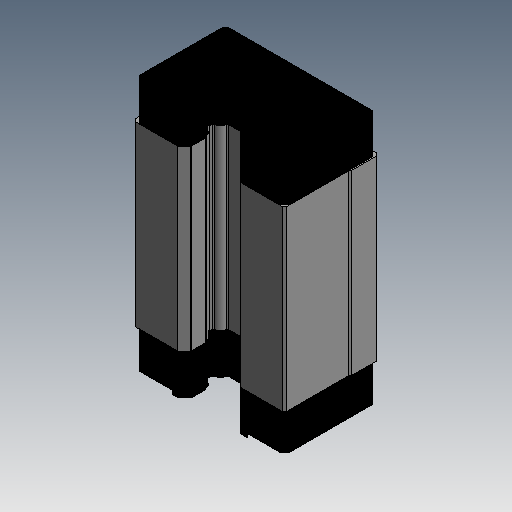
# Autodesk Inventor part: C-SXR24-R_b
Saved by Autodesk Inventor 2020 (Build 240168000, 168)
## iProperties
Part Number: C-SXR24-R_b
Material: 一般
Catalog Web Link: www.cadenas.de
Description: C-SXR, C-SX2R, C-SXRL, C-SX2RL_block-C-VALUE Linear Guides for Heavy Load
Vendor: MISUMI
Document SubType Name: Modeling
Designer: partserver
Manufacturer: MISUMI
Mass: 31.9411 g
Surface Area: 88.9166 cm^2
Volume: 31.9411 cm^3
Density: 1 g/cm^3
Appearance: PSOLRGB-192-192-192
Category: PARTsolutions
Company: MISUMI
PSOL_IDENT_0: {$CADENAS_DATA\23d-libs\misumi\metric\06_linear_guides\06_cn\c_sxr\c_sxr_block.prj},199 {VTYP=3D},{N
PSOL_IDENT_1: B=C-SXR24-R_b},{LINA=C-SXR24-R},{NN=C-SXR, C-SX2R, C-SXRL, C-SX2RL_block},{DATE=20.05.2021 06:43:21}
PSOL_IDENT_2: ,{GEOMDATE=17.04.2020 08:25:00},{VERSION=},{LINEID=10},{WBVAR=NOB,LT,BD},{WBNUMERIC=}  {NB=C-SXR24-R
PSOL_IDENT_3: _b},{LINA=C-SXR24-R},{KT=DUMMY},{PN=C-SXR24-R},{TYPE=C-SX},{H=24},{NOB=},{LT=},{W=34},{L1=55.9},{B=2
PSOL_IDENT_4: 6},{C=26},{SLL=M4x5},{S=4.000},{LL=5.000},{L2=39.5},{K=20.8},{T=6.20},{CBB=0.5},{E=7},{T1=5.5},{H1=1
PSOL_IDENT_5: 3.0},{W1=15},{W2=9.5},{CAA=0.5},{DD1=4.5},{DD2=7.5},{HH=6.0},{LW1=7.217},{LW2=11.000},{LH1=8.221},{L
PSOL_IDENT_6: H2=4.659},{LH3=3.221},{LH4=4.700},{LC1=0.300},{LC2=2.000},{LC3=0.500},{LR1=1.431},{LR2=0.300},{LR3=0
PSOL_IDENT_7: .300},{LR4=0.300},{BW=11.000},{BW2=33.400},{BH=20.250},{BH2=0.300},{BA1=149.392},{BA2=151.695},{CBB2=
PSOL_IDENT_8: 0.750},{CBB3=0.500},{CBB4=1.000},{HL=7.100},{BW3=7.105},{BW4=13.000},{BW5=17.000},{BW6=0.250},{BH3=1
PSOL_IDENT_9: 0.750},{BH4=2.417},{BH5=2.188},{BH6=0.500},{BA3=119.244},{BA4=131.813},{BA5=135.000},{BT=0.800},{BR=
PSOL_IDENT_10: 1.000},{BD=R}
NB: C-SXR24-R_b
NN: C-SXR, C-SX2R, C-SXRL, C-SX2RL_block
NT: C-VALUE Linear Guides for Heavy Load
NBSYN: $PN._b
LINA: C-SXR24-R
CATALOG: Misumi
PN: C-SXR24-R
H: 24
NOB: 1
LT: Selectable
W: 34
L1: 55.9
B: 26
C: 26
SLL: M4x5
L2: 39.5
K: 20.8
T: 6.2
CBB: 0.5
E: 7
T1: 5.5
BD: R
SUPPLIER: MISUMI
ARTICLENO: C-SXR24-R_b
BOMINFO: C-SXR24-R
CREATOR: CADENAS GmbH
Title: C-SXR24-R
Author: Cadenas PARTsolutions
Comments: C-VALUE Linear Guides for Heavy Load
Autodesk Inventor part; units mm, degrees
sketch "Sketch_1" plane through (0, 0, 0) normal (0, 0, 1) x (1, 0, 0)
  line L0 (-17, 23.5) -> (-17, 17.8)
  line L1 (-17, 17.8) -> (-16.75, 17.3358)
  line L2 (-16.75, 17.3358) -> (-16.75, 3.7)
  line L3 (-16.75, 3.7) -> (-16.25, 3.2)
  line L4 (-16.25, 3.2) -> (16.5, 3.2)
  line L5 (16.5, 3.2) -> (17, 3.7)
  line L6 (17, 3.7) -> (17, 23.5)
  line L7 (17, 23.5) -> (16.5, 24)
  line L8 (16.5, 24) -> (5.5, 24)
  line L9 (5.5, 24) -> (4.9929, 23.7)
  line L10 (4.9929, 23.7) -> (-4.9929, 23.7)
  line L11 (-4.9929, 23.7) -> (-5.5, 24)
  line L12 (-5.5, 24) -> (-16.5, 24)
  line L13 (-16.5, 24) -> (-17, 23.5)
  constraints: 28 end point
extrude "Extrusion1" add sketch "Sketch_1" along normal mid plane 39.5
sketch "Sketch_2" plane through (0, 0, 0) normal (0, 0, 1) x (1, 0, 0)
  line L0 (-16.7, 22.75) -> (-16.7, 4.3)
  line L1 (-16.7, 4.3) -> (-15.7, 3.3)
  line L2 (-15.7, 3.3) -> (15.7, 3.3)
  line L3 (15.7, 3.3) -> (16.7, 4.3)
  line L4 (16.7, 4.3) -> (16.7, 22.75)
  line L5 (16.7, 22.75) -> (15.95, 23.5)
  line L6 (15.95, 23.5) -> (-15.95, 23.5)
  line L7 (-15.95, 23.5) -> (-16.7, 22.75)
  constraints: 16 end point
extrude "Extrusion2" add sketch "Sketch_2" along normal mid plane 55.9
sketch "Sketch_32" plane through (0, 18.5, 0) normal (0, 1, 0) x (1, 0, 0)
  line L0 (0, -27.95) -> (0, -34.95)
  arc A0 (-3, -31.95) -> (0, -34.95) centre (0, -31.95) ccw
  line L1 (-3, -31.95) -> (-3, -27.95)
  line L2 (-3, -27.95) -> (0, -27.95)
  line L3 (0, -27.95) -> (0, -34.95)
  constraints: 8 end point, 2 point on circle, 1 centre point
revolve "Revolution1" add sketch "Sketch_32" angle 360 about axis through (0, 18.5, 27.95) along (0, 0, -1)
sketch "Sketch_33" plane through (0, 0, 27.95) normal (0, 0, 1) x (1, 0, 0)
  circle A0 centre (0, 18.5) radius 3.5
  line L0 (-2.8868, 18.5) -> (-1.4434, 16)
  line L1 (-1.4434, 16) -> (1.4434, 16)
  line L2 (1.4434, 16) -> (2.8868, 18.5)
  line L3 (2.8868, 18.5) -> (1.4434, 21)
  line L4 (1.4434, 21) -> (-1.4434, 21)
  line L5 (-1.4434, 21) -> (-2.8868, 18.5)
  constraints: 12 end point, 1 centre point
extrude "Extrusion3" cut sketch "Sketch_33" along normal blind 7
sketch "Sketch_7" plane through (0, 0, 27.95) normal (0, 0, 1) x (1, 0, 0)
  line L0 (-8.5, 11.2475) -> (-8.5, 9.5386)
  arc A0 (-8.5, 9.5386) -> (-8.1667, 8.7933) centre (-7.5, 9.5386) ccw
  line L1 (-8.1667, 8.7933) -> (-6.8333, 7.6006)
  arc A1 (-6.5, 6.8552) -> (-6.8333, 7.6006) centre (-7.5, 6.8552) ccw
  line L2 (-6.5, 6.8552) -> (-6.5, 5.5286)
  arc A2 (-6.7929, 4.8215) -> (-6.5, 5.5286) centre (-7.5, 5.5286) ccw
  line L3 (-6.7929, 4.8215) -> (-8.3144, 3.3)
  line L4 (-8.3144, 3.3) -> (8.3144, 3.3)
  line L5 (8.3144, 3.3) -> (6.7929, 4.8215)
  arc A3 (6.5, 5.5286) -> (6.7929, 4.8215) centre (7.5, 5.5286) ccw
  line L6 (6.5, 5.5286) -> (6.5, 6.8552)
  arc A4 (6.8333, 7.6006) -> (6.5, 6.8552) centre (7.5, 6.8552) ccw
  line L7 (6.8333, 7.6006) -> (8.1667, 8.7933)
  arc A5 (8.1667, 8.7933) -> (8.5, 9.5386) centre (7.5, 9.5386) ccw
  line L8 (8.5, 9.5386) -> (8.5, 11.2475)
  arc A6 (8.5, 11.2475) -> (8.3725, 11.7361) centre (7.5, 11.2475) ccw
  line L9 (8.3725, 11.7361) -> (7.3914, 13.4885)
  arc A7 (7.3914, 13.4885) -> (6.5188, 14) centre (6.5188, 13) ccw
  line L10 (6.5188, 14) -> (-6.5188, 14)
  arc A8 (-6.5188, 14) -> (-7.3914, 13.4885) centre (-6.5188, 13) ccw
  line L11 (-7.3914, 13.4885) -> (-8.3725, 11.7361)
  arc A9 (-8.3725, 11.7361) -> (-8.5, 11.2475) centre (-7.5, 11.2475) ccw
  constraints: 24 end point, 20 point on circle, 10 centre point
extrude "Extrusion4" add sketch "Sketch_7" along normal blind 0.8
sketch "Sketch_47" plane through (0, 0, -27.95) normal (0, 0, 1) x (1, 0, 0)
  line L0 (-8.5, 11.2475) -> (-8.5, 9.5386)
  arc A0 (-8.5, 9.5386) -> (-8.1667, 8.7933) centre (-7.5, 9.5386) ccw
  line L1 (-8.1667, 8.7933) -> (-6.8333, 7.6006)
  arc A1 (-6.5, 6.8552) -> (-6.8333, 7.6006) centre (-7.5, 6.8552) ccw
  line L2 (-6.5, 6.8552) -> (-6.5, 5.5286)
  arc A2 (-6.7929, 4.8215) -> (-6.5, 5.5286) centre (-7.5, 5.5286) ccw
  line L3 (-6.7929, 4.8215) -> (-8.3144, 3.3)
  line L4 (-8.3144, 3.3) -> (8.3144, 3.3)
  line L5 (8.3144, 3.3) -> (6.7929, 4.8215)
  arc A3 (6.5, 5.5286) -> (6.7929, 4.8215) centre (7.5, 5.5286) ccw
  line L6 (6.5, 5.5286) -> (6.5, 6.8552)
  arc A4 (6.8333, 7.6006) -> (6.5, 6.8552) centre (7.5, 6.8552) ccw
  line L7 (6.8333, 7.6006) -> (8.1667, 8.7933)
  arc A5 (8.1667, 8.7933) -> (8.5, 9.5386) centre (7.5, 9.5386) ccw
  line L8 (8.5, 9.5386) -> (8.5, 11.2475)
  arc A6 (8.5, 11.2475) -> (8.3725, 11.7361) centre (7.5, 11.2475) ccw
  line L9 (8.3725, 11.7361) -> (7.3914, 13.4885)
  arc A7 (7.3914, 13.4885) -> (6.5188, 14) centre (6.5188, 13) ccw
  line L10 (6.5188, 14) -> (-6.5188, 14)
  arc A8 (-6.5188, 14) -> (-7.3914, 13.4885) centre (-6.5188, 13) ccw
  line L11 (-7.3914, 13.4885) -> (-8.3725, 11.7361)
  arc A9 (-8.3725, 11.7361) -> (-8.5, 11.2475) centre (-7.5, 11.2475) ccw
  constraints: 24 end point, 20 point on circle, 10 centre point
extrude "Extrusion5" add sketch "Sketch_47" against normal blind 0.8
sketch "Sketch_3" plane through (0, 0, 0) normal (0, 0, 1) x (1, 0, 0)
  line L0 (-7.5, 10.787) -> (-7.5, 10.313)
  line L1 (-7.5, 10.313) -> (-7.2658, 9.8108)
  arc A0 (-7.2658, 9.8108) -> (-7.0326, 9.6401) centre (-6.9939, 9.9376) ccw
  arc A1 (-5.7891, 8.3153) -> (-7.0326, 9.6401) centre (-7.217, 8.221) ccw
  arc A2 (-5.7891, 8.3153) -> (-5.7019, 8.1229) centre (-5.4898, 8.335) ccw
  line L2 (-5.7019, 8.1229) -> (-5.5879, 8.0089)
  arc A3 (-5.5, 7.7967) -> (-5.5879, 8.0089) centre (-5.8, 7.7967) ccw
  line L3 (-5.5, 7.7967) -> (-5.5, 4.8243)
  arc A4 (-5.5879, 4.6121) -> (-5.5, 4.8243) centre (-5.8, 4.8243) ccw
  line L4 (-5.5879, 4.6121) -> (-7.4121, 2.7879)
  arc A5 (-7.4121, 2.7879) -> (-7.5, 2.5757) centre (-7.2, 2.5757) ccw
  line L5 (-7.5, 2.5757) -> (-7.5, 0.5)
  line L6 (-7.5, 0.5) -> (-7, 0)
  line L7 (-7, 0) -> (7, 0)
  line L8 (7, 0) -> (7.5, 0.5)
  line L9 (7.5, 0.5) -> (7.5, 2.5757)
  arc A6 (7.5, 2.5757) -> (7.4121, 2.7879) centre (7.2, 2.5757) ccw
  line L10 (7.4121, 2.7879) -> (5.5879, 4.6121)
  arc A7 (5.5, 4.8243) -> (5.5879, 4.6121) centre (5.8, 4.8243) ccw
  line L11 (5.5, 4.8243) -> (5.5, 7.7967)
  arc A8 (5.5879, 8.0089) -> (5.5, 7.7967) centre (5.8, 7.7967) ccw
  line L12 (5.5879, 8.0089) -> (5.7019, 8.1229)
  arc A9 (5.7019, 8.1229) -> (5.7891, 8.3153) centre (5.4898, 8.335) ccw
  arc A10 (7.0326, 9.6401) -> (5.7891, 8.3153) centre (7.217, 8.221) ccw
  arc A11 (7.0326, 9.6401) -> (7.2658, 9.8108) centre (6.9939, 9.9376) ccw
  line L13 (7.2658, 9.8108) -> (7.5, 10.313)
  line L14 (7.5, 10.313) -> (7.5, 10.787)
  line L15 (7.5, 10.787) -> (7.2653, 11.2903)
  arc A12 (7.2653, 11.2903) -> (7.0322, 11.461) centre (6.9934, 11.1635) ccw
  arc A13 (5.7938, 12.7312) -> (7.0322, 11.461) centre (7.217, 12.88) ccw
  arc A14 (5.7938, 12.7312) -> (5.4954, 13) centre (5.4954, 12.7) ccw
  line L16 (5.4954, 13) -> (-5.4954, 13)
  arc A15 (-5.4954, 13) -> (-5.7938, 12.7312) centre (-5.4954, 12.7) ccw
  arc A16 (-7.0322, 11.461) -> (-5.7938, 12.7312) centre (-7.217, 12.88) ccw
  arc A17 (-7.0322, 11.461) -> (-7.2653, 11.2903) centre (-6.9934, 11.1635) ccw
  line L17 (-7.2653, 11.2903) -> (-7.5, 10.787)
  constraints: 36 end point, 36 point on circle, 18 centre point
extrude "Extrusion6" cut sketch "Sketch_3" along normal mid plane 39.5
sketch "Sketch_11" plane through (0, 0, 19.75) normal (0, 0, 1) x (1, 0, 0)
  line L0 (-7.5, 10.787) -> (-7.5, 10.313)
  line L1 (-7.5, 10.313) -> (-7.2658, 9.8108)
  arc A0 (-7.2658, 9.8108) -> (-7.0326, 9.6401) centre (-6.9939, 9.9376) ccw
  arc A1 (-5.7891, 8.3153) -> (-7.0326, 9.6401) centre (-7.217, 8.221) ccw
  arc A2 (-5.7891, 8.3153) -> (-5.7019, 8.1229) centre (-5.4898, 8.335) ccw
  line L2 (-5.7019, 8.1229) -> (-5.5879, 8.0089)
  arc A3 (-5.5, 7.7967) -> (-5.5879, 8.0089) centre (-5.8, 7.7967) ccw
  line L3 (-5.5, 7.7967) -> (-5.5, 4.8243)
  arc A4 (-5.5879, 4.6121) -> (-5.5, 4.8243) centre (-5.8, 4.8243) ccw
  line L4 (-5.5879, 4.6121) -> (-7.4121, 2.7879)
  arc A5 (-7.4121, 2.7879) -> (-7.5, 2.5757) centre (-7.2, 2.5757) ccw
  line L5 (-7.5, 2.5757) -> (-7.5, 0.5)
  line L6 (-7.5, 0.5) -> (-7, 0)
  line L7 (-7, 0) -> (7, 0)
  line L8 (7, 0) -> (7.5, 0.5)
  line L9 (7.5, 0.5) -> (7.5, 2.5757)
  arc A6 (7.5, 2.5757) -> (7.4121, 2.7879) centre (7.2, 2.5757) ccw
  line L10 (7.4121, 2.7879) -> (5.5879, 4.6121)
  arc A7 (5.5, 4.8243) -> (5.5879, 4.6121) centre (5.8, 4.8243) ccw
  line L11 (5.5, 4.8243) -> (5.5, 7.7967)
  arc A8 (5.5879, 8.0089) -> (5.5, 7.7967) centre (5.8, 7.7967) ccw
  line L12 (5.5879, 8.0089) -> (5.7019, 8.1229)
  arc A9 (5.7019, 8.1229) -> (5.7891, 8.3153) centre (5.4898, 8.335) ccw
  arc A10 (7.0326, 9.6401) -> (5.7891, 8.3153) centre (7.217, 8.221) ccw
  arc A11 (7.0326, 9.6401) -> (7.2658, 9.8108) centre (6.9939, 9.9376) ccw
  line L13 (7.2658, 9.8108) -> (7.5, 10.313)
  line L14 (7.5, 10.313) -> (7.5, 10.787)
  line L15 (7.5, 10.787) -> (7.2653, 11.2903)
  arc A12 (7.2653, 11.2903) -> (7.0322, 11.461) centre (6.9934, 11.1635) ccw
  arc A13 (5.7938, 12.7312) -> (7.0322, 11.461) centre (7.217, 12.88) ccw
  arc A14 (5.7938, 12.7312) -> (5.4954, 13) centre (5.4954, 12.7) ccw
  line L16 (5.4954, 13) -> (-5.4954, 13)
  arc A15 (-5.4954, 13) -> (-5.7938, 12.7312) centre (-5.4954, 12.7) ccw
  arc A16 (-7.0322, 11.461) -> (-5.7938, 12.7312) centre (-7.217, 12.88) ccw
  arc A17 (-7.0322, 11.461) -> (-7.2653, 11.2903) centre (-6.9934, 11.1635) ccw
  line L17 (-7.2653, 11.2903) -> (-7.5, 10.787)
  constraints: 36 end point, 36 point on circle, 18 centre point
extrude "Extrusion7" cut sketch "Sketch_11" along normal blind 19.75
sketch "Sketch_12" plane through (0, 0, -19.75) normal (0, 0, 1) x (1, 0, 0)
  line L0 (-7.5, 10.787) -> (-7.5, 10.313)
  line L1 (-7.5, 10.313) -> (-7.2658, 9.8108)
  arc A0 (-7.2658, 9.8108) -> (-7.0326, 9.6401) centre (-6.9939, 9.9376) ccw
  arc A1 (-5.7891, 8.3153) -> (-7.0326, 9.6401) centre (-7.217, 8.221) ccw
  arc A2 (-5.7891, 8.3153) -> (-5.7019, 8.1229) centre (-5.4898, 8.335) ccw
  line L2 (-5.7019, 8.1229) -> (-5.5879, 8.0089)
  arc A3 (-5.5, 7.7967) -> (-5.5879, 8.0089) centre (-5.8, 7.7967) ccw
  line L3 (-5.5, 7.7967) -> (-5.5, 4.8243)
  arc A4 (-5.5879, 4.6121) -> (-5.5, 4.8243) centre (-5.8, 4.8243) ccw
  line L4 (-5.5879, 4.6121) -> (-7.4121, 2.7879)
  arc A5 (-7.4121, 2.7879) -> (-7.5, 2.5757) centre (-7.2, 2.5757) ccw
  line L5 (-7.5, 2.5757) -> (-7.5, 0.5)
  line L6 (-7.5, 0.5) -> (-7, 0)
  line L7 (-7, 0) -> (7, 0)
  line L8 (7, 0) -> (7.5, 0.5)
  line L9 (7.5, 0.5) -> (7.5, 2.5757)
  arc A6 (7.5, 2.5757) -> (7.4121, 2.7879) centre (7.2, 2.5757) ccw
  line L10 (7.4121, 2.7879) -> (5.5879, 4.6121)
  arc A7 (5.5, 4.8243) -> (5.5879, 4.6121) centre (5.8, 4.8243) ccw
  line L11 (5.5, 4.8243) -> (5.5, 7.7967)
  arc A8 (5.5879, 8.0089) -> (5.5, 7.7967) centre (5.8, 7.7967) ccw
  line L12 (5.5879, 8.0089) -> (5.7019, 8.1229)
  arc A9 (5.7019, 8.1229) -> (5.7891, 8.3153) centre (5.4898, 8.335) ccw
  arc A10 (7.0326, 9.6401) -> (5.7891, 8.3153) centre (7.217, 8.221) ccw
  arc A11 (7.0326, 9.6401) -> (7.2658, 9.8108) centre (6.9939, 9.9376) ccw
  line L13 (7.2658, 9.8108) -> (7.5, 10.313)
  line L14 (7.5, 10.313) -> (7.5, 10.787)
  line L15 (7.5, 10.787) -> (7.2653, 11.2903)
  arc A12 (7.2653, 11.2903) -> (7.0322, 11.461) centre (6.9934, 11.1635) ccw
  arc A13 (5.7938, 12.7312) -> (7.0322, 11.461) centre (7.217, 12.88) ccw
  arc A14 (5.7938, 12.7312) -> (5.4954, 13) centre (5.4954, 12.7) ccw
  line L16 (5.4954, 13) -> (-5.4954, 13)
  arc A15 (-5.4954, 13) -> (-5.7938, 12.7312) centre (-5.4954, 12.7) ccw
  arc A16 (-7.0322, 11.461) -> (-5.7938, 12.7312) centre (-7.217, 12.88) ccw
  arc A17 (-7.0322, 11.461) -> (-7.2653, 11.2903) centre (-6.9934, 11.1635) ccw
  line L17 (-7.2653, 11.2903) -> (-7.5, 10.787)
  constraints: 36 end point, 36 point on circle, 18 centre point
extrude "Extrusion8" cut sketch "Sketch_12" against normal blind 19.75
sketch "Sketch10" plane through (5.5, 24, 19.75) normal (0, 1, 0) x (1, 0, 0)
  point P0 (7.5, 6.75)
hole "Hole1" at (13, 24, 13) direction (0, -1, 0) diameter 3.242 depth 7.1 tip angle 120 countersink diameter 4 countersink angle 90 thread size "M4x0.7" class "6H" standard "ISO Metric profile"
pattern_linear "Rectangular Pattern1" count 2 spacing 26 along (0, 0, -1) count 2 spacing 26 along (-1, 0, 0) of "Hole1"
sketch "Sketch_29" plane through (0, 0, 19.75) normal (0, 0, 1) x (1, 0, 0)
  line L0 (-7.55, 0.5) -> (-7.05, 0)
  line L1 (-7.05, 0) -> (7.05, 0)
  line L2 (7.05, 0) -> (7.55, 0.5)
  line L3 (7.55, 0.5) -> (7.55, 2.6017)
  arc A0 (7.55, 2.6017) -> (7.4477, 2.849) centre (7.2, 2.6017) ccw
  line L4 (7.4477, 2.849) -> (5.6523, 4.6475)
  arc A1 (5.55, 4.8948) -> (5.6523, 4.6475) centre (5.9, 4.8948) ccw
  line L5 (5.55, 4.8948) -> (5.55, 7.7762)
  arc A2 (5.6523, 8.0235) -> (5.55, 7.7762) centre (5.9, 7.7762) ccw
  line L6 (5.6523, 8.0235) -> (5.6888, 8.06)
  arc A3 (5.6888, 8.06) -> (5.7901, 8.2812) centre (5.4411, 8.3073) ccw
  arc A4 (7.0392, 9.6344) -> (5.7901, 8.2812) centre (7.267, 8.171) ccw
  arc A5 (7.0392, 9.6344) -> (7.3025, 9.8323) centre (6.9853, 9.9802) ccw
  line L7 (7.3025, 9.8323) -> (7.55, 10.363)
  line L8 (7.55, 10.363) -> (7.55, 10.887)
  line L9 (7.55, 10.887) -> (7.3767, 11.2587)
  arc A6 (7.3767, 11.2587) -> (7.0991, 11.4585) centre (7.0595, 11.1108) ccw
  arc A7 (5.7977, 12.744) -> (7.0991, 11.4585) centre (7.267, 12.93) ccw
  arc A8 (5.7977, 12.744) -> (5.4505, 13.05) centre (5.4505, 12.7) ccw
  line L10 (5.4505, 13.05) -> (-5.4505, 13.05)
  arc A9 (-5.4505, 13.05) -> (-5.7977, 12.744) centre (-5.4505, 12.7) ccw
  arc A10 (-7.0991, 11.4585) -> (-5.7977, 12.744) centre (-7.267, 12.93) ccw
  arc A11 (-7.0991, 11.4585) -> (-7.3767, 11.2587) centre (-7.0595, 11.1108) ccw
  line L11 (-7.3767, 11.2587) -> (-7.55, 10.887)
  line L12 (-7.55, 10.887) -> (-7.55, 10.363)
  line L13 (-7.55, 10.363) -> (-7.3025, 9.8323)
  arc A12 (-7.3025, 9.8323) -> (-7.0392, 9.6344) centre (-6.9853, 9.9802) ccw
  arc A13 (-5.7901, 8.2812) -> (-7.0392, 9.6344) centre (-7.267, 8.171) ccw
  arc A14 (-5.7901, 8.2812) -> (-5.6888, 8.06) centre (-5.4411, 8.3073) ccw
  line L14 (-5.6888, 8.06) -> (-5.6523, 8.0235)
  arc A15 (-5.55, 7.7762) -> (-5.6523, 8.0235) centre (-5.9, 7.7762) ccw
  line L15 (-5.55, 7.7762) -> (-5.55, 4.8948)
  arc A16 (-5.6523, 4.6475) -> (-5.55, 4.8948) centre (-5.9, 4.8948) ccw
  line L16 (-5.6523, 4.6475) -> (-7.4477, 2.849)
  arc A17 (-7.4477, 2.849) -> (-7.55, 2.6017) centre (-7.2, 2.6017) ccw
  line L17 (-7.55, 2.6017) -> (-7.55, 0.5)
  constraints: 36 end point, 36 point on circle, 18 centre point
extrude "Extrusion9" cut sketch "Sketch_29" along normal blind 0.05
sketch "Sketch_30" plane through (0, 0, -19.75) normal (0, 0, 1) x (1, 0, 0)
  line L0 (-7.55, 0.5) -> (-7.05, 0)
  line L1 (-7.05, 0) -> (7.05, 0)
  line L2 (7.05, 0) -> (7.55, 0.5)
  line L3 (7.55, 0.5) -> (7.55, 2.6017)
  arc A0 (7.55, 2.6017) -> (7.4477, 2.849) centre (7.2, 2.6017) ccw
  line L4 (7.4477, 2.849) -> (5.6523, 4.6475)
  arc A1 (5.55, 4.8948) -> (5.6523, 4.6475) centre (5.9, 4.8948) ccw
  line L5 (5.55, 4.8948) -> (5.55, 7.7762)
  arc A2 (5.6523, 8.0235) -> (5.55, 7.7762) centre (5.9, 7.7762) ccw
  line L6 (5.6523, 8.0235) -> (5.6888, 8.06)
  arc A3 (5.6888, 8.06) -> (5.7901, 8.2812) centre (5.4411, 8.3073) ccw
  arc A4 (7.0392, 9.6344) -> (5.7901, 8.2812) centre (7.267, 8.171) ccw
  arc A5 (7.0392, 9.6344) -> (7.3025, 9.8323) centre (6.9853, 9.9802) ccw
  line L7 (7.3025, 9.8323) -> (7.55, 10.363)
  line L8 (7.55, 10.363) -> (7.55, 10.887)
  line L9 (7.55, 10.887) -> (7.3767, 11.2587)
  arc A6 (7.3767, 11.2587) -> (7.0991, 11.4585) centre (7.0595, 11.1108) ccw
  arc A7 (5.7977, 12.744) -> (7.0991, 11.4585) centre (7.267, 12.93) ccw
  arc A8 (5.7977, 12.744) -> (5.4505, 13.05) centre (5.4505, 12.7) ccw
  line L10 (5.4505, 13.05) -> (-5.4505, 13.05)
  arc A9 (-5.4505, 13.05) -> (-5.7977, 12.744) centre (-5.4505, 12.7) ccw
  arc A10 (-7.0991, 11.4585) -> (-5.7977, 12.744) centre (-7.267, 12.93) ccw
  arc A11 (-7.0991, 11.4585) -> (-7.3767, 11.2587) centre (-7.0595, 11.1108) ccw
  line L11 (-7.3767, 11.2587) -> (-7.55, 10.887)
  line L12 (-7.55, 10.887) -> (-7.55, 10.363)
  line L13 (-7.55, 10.363) -> (-7.3025, 9.8323)
  arc A12 (-7.3025, 9.8323) -> (-7.0392, 9.6344) centre (-6.9853, 9.9802) ccw
  arc A13 (-5.7901, 8.2812) -> (-7.0392, 9.6344) centre (-7.267, 8.171) ccw
  arc A14 (-5.7901, 8.2812) -> (-5.6888, 8.06) centre (-5.4411, 8.3073) ccw
  line L14 (-5.6888, 8.06) -> (-5.6523, 8.0235)
  arc A15 (-5.55, 7.7762) -> (-5.6523, 8.0235) centre (-5.9, 7.7762) ccw
  line L15 (-5.55, 7.7762) -> (-5.55, 4.8948)
  arc A16 (-5.6523, 4.6475) -> (-5.55, 4.8948) centre (-5.9, 4.8948) ccw
  line L16 (-5.6523, 4.6475) -> (-7.4477, 2.849)
  arc A17 (-7.4477, 2.849) -> (-7.55, 2.6017) centre (-7.2, 2.6017) ccw
  line L17 (-7.55, 2.6017) -> (-7.55, 0.5)
  constraints: 36 end point, 36 point on circle, 18 centre point
extrude "Extrusion10" cut sketch "Sketch_30" against normal blind 0.05
ref_plane "to_rail_XY" through (0, 13, 0) normal (0, 0, 1) x (1, 0, 0)
ref_plane "to_rail_YZ" through (0, 13, 0) normal (1, 0, 0) x (0, 1, 0)
ref_plane "to_rail_ZX" through (0, 13, 0) normal (0, 1, 0) x (0, 0, 1)
body "Solid1"
